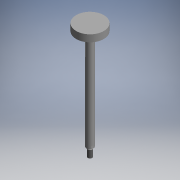
# Autodesk Inventor part: 1808236 DFPI-100-280-ND2P-E-P(K)
Saved by Autodesk Inventor 2017.3 (Build 213256000, 256)
## iProperties
Part Number: 1808236 DFPI-100-280-ND2P-E-P(K)
Material: Generic
Catalog Web Link: www.cadenas.de
Description: DFPI_KOLBEN-Linear drive - piston
Vendor: FESTO
Document SubType Name: Modeling
Designer: partserver
Manufacturer: FESTO
Mass: 379.963 g
Surface Area: 535.794 cm^2
Volume: 379.963 cm^3
Density: 1 g/cm^3
Appearance: PSOLRGB-192-192-192
Category: PARTsolutions
Company: FESTO
Title: 1808236 DFPI-100-280-ND2P-E-P(K)
Author: Cadenas PARTsolutions
Comments: Linear drive - piston
PSOL_IDENT_0: {$CADENAS_DATA\23d-libs\festo\parts\d\dfpi\parts\dfpi_ep_kolben.prj},216 {VTYP=3D},{NB=1808236 DFPI-
PSOL_IDENT_1: 100-280-ND2P-E-P(K)},{LINA=1808236 DFPI-100-280-ND2P-E-P(K)},{NN=DFPI_KOLBEN},{DATE=14.05.2021 07:20
PSOL_IDENT_2: :23},{GEOMDATE=20.07.2016 06:08:00},{VERSION=},{LINEID=250},{WBVAR=HUB},{WBNUMERIC=HUB}  {NB=1808236
PSOL_IDENT_3: DFPI-100-280-ND2P-E-P(K)},{LINA=1808236 DFPI-100-280-ND2P-E-P(K)},{KT=DUMMY},{TNR=1808236},{TYP=DFP
PSOL_IDENT_4: I},{TYP2=DFPI-100-    -ND2P-E-P-G2},{HUB=280},{KDM=100},{DF=N},{WS=D2},{MF=P},{RE=-},{RE1=},{AR=E},{
PSOL_IDENT_5: AR1=-E},{WV=-},{WV1=},{AF=P},{AF1=-P},{RM=-},{RM1=},{L0=118.500},{AM=32.000},{D2=25.000},{KK=M16x1.5
PSOL_IDENT_6: },{KKNDM=16.000},{KKP=1.500},{SW1=22.000},{WH=16.000},{L100=27.500},{L101=10.000},{DG=13.000},{G1=2.
PSOL_IDENT_7: 500},{G2=5.000},{R=1.000},{CH=0.400},{VERS=19}
NB: 1808236 DFPI-100-280-ND2P-E-P(K)
NN: DFPI_KOLBEN
NT: Linear drive - piston
NBSYN: $TNR. $TYP.-$KDM.-$HUB.-$DF.$WS.$MF.$RE1.$AR1.$WV1.$AF1.$RM1.(K)
LINA: 1808236 DFPI-100-280-ND2P-E-P(K)
CATALOG: Festo
TNR: 1808236
TYP: DFPI
TYP2: DFPI-100-    -ND2P-E-P-G2
HUB: 280
KDM: 100
DF: N
WS: D2
MF: P
RE: -
AR: E
WV: -
AF: P
RM: -
L0: 118.5
AM: 32
D2: 25
KK: M16x1.5
KKNDM: 16
KKP: 1.5
SW1: 22
WH: 16
L100: 27.5
L101: 10
DG: 13
G1: 2.5
G2: 5
R: 1
CH: 0.4
VERS: 19
SUPPLIER: FESTO
ARTICLENO: 1808236 DFPI-100-280-ND2P-E-P(K)
BOMINFO: 1808236 DFPI-100-280-ND2P-E-P(K)
CREATOR: CADENAS GmbH
Autodesk Inventor part; units mm, degrees
sketch "Sketch_1" plane through (0, 0, 0) normal (1, 0, 0) x (0, 1, 0)
  line L0 (0, -387) -> (0, 0)
  line L1 (0, 0) -> (12.1, 0)
  line L2 (12.1, 0) -> (12.5, -0.4)
  line L3 (12.5, -0.4) -> (12.5, -362)
  line L4 (12.5, -362) -> (50, -362)
  line L5 (50, -362) -> (50, -387)
  line L6 (50, -387) -> (0, -387)
  line L7 (0, -387) -> (0, 0)
  constraints: 16 end point
revolve "Revolution1" add sketch "Sketch_1" angle 360 about axis through (0, 0, -387) along (0, 0, -1)
sketch "Sketch_2" plane through (0, 0, 0) normal (1, 0, 0) x (0, 1, 0)
  line L0 (0, -1) -> (0, 32)
  line L1 (0, 32) -> (7.08, 32)
  line L2 (7.08, 32) -> (8, 31.08)
  line L3 (8, 31.08) -> (8, 5)
  line L4 (8, 5) -> (6.6425, 2.7375)
  arc A0 (6.6425, 2.7375) -> (6.5, 2.223) centre (7.5, 2.223) ccw
  line L5 (6.5, 2.223) -> (6.5, 1)
  arc A1 (6.5, 1) -> (7.5, 0) centre (7.5, 1) ccw
  line L6 (7.5, 0) -> (8, 0)
  line L7 (8, 0) -> (8, -1)
  line L8 (8, -1) -> (0, -1)
  line L9 (0, -1) -> (0, 32)
  constraints: 20 end point, 4 point on circle, 2 centre point
revolve "Revolution2" add sketch "Sketch_2" angle 360 about axis through (0, 0, -1) along (0, 0, -1)
thread "Thread1" size "M16x1.5" class "6g" standard "ISO Metric profile" full length
sketch "Sketch_4" plane through (0, 0, 0) normal (0, 1, 0) x (-1, 0, 0)
  line L0 (15.5, -10.4) -> (15.5, 36.6)
  line L1 (15.5, 36.6) -> (-15.5, 36.6)
  line L2 (-15.5, 36.6) -> (-15.5, -10.4)
  line L3 (-15.5, -10.4) -> (-11, -10.4)
  line L4 (-11, -10.4) -> (-11, 0)
  line L5 (-11, 0) -> (-14.5, 0)
  line L6 (-14.5, 0) -> (-14.5, 35.6)
  line L7 (-14.5, 35.6) -> (14.5, 35.6)
  line L8 (14.5, 35.6) -> (14.5, 0)
  line L9 (14.5, 0) -> (11, 0)
  line L10 (11, 0) -> (11, -10.4)
  line L11 (11, -10.4) -> (15.5, -10.4)
  constraints: 24 end point
extrude "Extrusion1" cut sketch "Sketch_4" along normal mid plane 25
sketch "Sketch_5" plane through (0, 0, 0) normal (0, 1, 0) x (-1, 0, 0)
  line L0 (0, -10) -> (0, -10.4)
  line L1 (0, -10.4) -> (-12.5, -10.4)
  line L2 (-12.5, -10.4) -> (-12.1, -10)
  line L3 (-12.1, -10) -> (0, -10)
  line L4 (0, -10) -> (0, -10.4)
  constraints: 10 end point
revolve "Revolution3" add sketch "Sketch_5" angle 360 about axis through (0, 0, -10) along (0, 0, 1)
ref_plane "KOLBEN_XY" through (0, 0, -387) normal (0, 0, -1) x (1, 0, 0)
ref_plane "KOLBEN_YZ" through (0, 0, -387) normal (1, 0, 0) x (0, -1, 0)
ref_plane "KOLBEN_ZX" through (0, 0, -387) normal (0, -1, 0) x (0, 0, -1)
body "Solid1"
